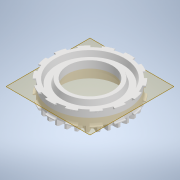
# Autodesk Inventor part: CAT_slave_wheel
Saved by Autodesk Inventor 2022 (Build 260153000, 153)
## iProperties
Created: 2024-07-28
Part Number: CAT_slave_wheel
Material: Типовые
Document SubType Name: Modeling
Designer: Капустяник Андрей
Density: 1 g/cm^3
Appearance: По умолчанию
Author: Капустяник Андрей
Autodesk Inventor part; units mm, degrees
ref_plane "YZ Plane" through (0, 0, 0) normal (1, 0, 0) x (0, 1, 0)
ref_plane "XZ Plane" through (0, 0, 0) normal (0, 1, 0) x (-1, 0, 0)
ref_plane "XY Plane" through (0, 0, 0) normal (0, 0, 1) x (1, 0, 0)
sketch "Эскиз1" plane through (0, 0, 0) normal (0, 1, 0) x (-1, 0, 0)
  circle A0 centre (0, 0) radius 35
  circle A1 centre (0, 0) radius 32
  circle A2 centre (0, 0) radius 18.5
  circle A3 centre (0, 0) radius 12.625
  circle A4 centre (0, 0) radius 18.6
  dimension "d0" = 70
  dimension "d1" = 3
  dimension "d2" = 37
  dimension "d3" = 25.25
  dimension "d4" = 37.2
  constraints: 5 centre point, 4 coincident
  measures "d0" diameter of A0
  measures "d1" radial gap between concentric circles of A0 A1
  measures "d2" diameter of A2
  measures "d3" diameter of A3
  measures "d4" diameter of A4
extrude "Выдавливание1" add sketch "Эскиз1" along normal blind 12 contours A1
sketch "Эскиз2" plane through (0, 0, 0) normal (0, -1, 0) x (1, 0, 0)
  circle A0 centre (0, 0) radius 32 projected
  circle A1 centre (0, 0) radius 18.6 projected
  circle A2 centre (-11.1467, 16) radius 3.5 projected
  circle A3 centre (-11.1467, 16) radius 6.5
  circle A4 centre (0, 0) radius 26
  dimension "d7" = 13
  constraints: 2 centre point, 2 coincident, 1 tangent
  measures "d7" diameter of A3
extrude "Выдавливание2" cut sketch "Эскиз2" against normal blind 5 contours A4 | A1 A2 A3 | A1 A2 picked at (-14.6701, 20.1761) picked at (-11.4582, 16.4471)
sketch "Эскиз3" plane through (0, 0, 0) normal (0, -1, 0) x (1, 0, 0)
  circle A0 centre (0, 0) radius 26
  circle A1 centre (0, 0) radius 32
  circle A2 centre (0, 0) radius 26
  circle A3 centre (0, 0) radius 18.6
  circle A4 centre (0, 0) radius 30
  spline S0 degree 3 poles (-0.9532, 24.4021) (-0.9433, 24.442) (-0.9236, 24.5218) (-0.8805, 24.6804) (-0.822, 24.8775) (-0.7447, 25.1117) (-0.661, 25.3437) (-0.5713, 25.5734) (-0.4759, 25.8008) (-0.3757, 26.0262) (-0.3047, 26.1745) (-0.2692, 26.2486) knots 0 0 0 0 0.062501 0.125002 0.25 0.374999 0.499998 0.624998 0.749999 0.875 1 1 1 1
  spline S1 degree 3 poles (0.9532, 24.4021) (0.9433, 24.442) (0.9236, 24.5218) (0.8805, 24.6804) (0.822, 24.8775) (0.7447, 25.1117) (0.661, 25.3437) (0.5713, 25.5734) (0.4759, 25.8008) (0.3757, 26.0262) (0.3047, 26.1745) (0.2692, 26.2486) knots 0 0 0 0 0.062501 0.125002 0.25 0.374999 0.499998 0.624998 0.749999 0.875 1 1 1 1
  circle A5 centre (0, 0) radius 26.25 construction
  circle A6 centre (0, 0) radius 23.4923 construction
  circle A7 centre (0, 0) radius 25 construction
  circle A8 centre (0, 0) radius 24.4207
  circle A9 centre (0, 0) radius 28.0793
  arc A10 (0.2692, 26.2486) -> (-0.2692, 26.2486) centre (0, 0) ccw
  point P0 (-0.9231, 24.5217)
  point P1 (-0.891, 24.6407)
  point P2 (-0.8208, 24.8771)
  point P3 (-0.7436, 25.1113)
  point P4 (-0.66, 25.3433)
  point P5 (-0.5703, 25.573)
  point P6 (-0.4751, 25.8005)
  point P7 (-0.3747, 26.0257)
  point P8 (0.9231, 24.5217)
  point P9 (0.891, 24.6407)
  point P10 (0.8208, 24.8771)
  point P11 (0.7436, 25.1113)
  point P12 (0.66, 25.3433)
  point P13 (0.5703, 25.573)
  point P14 (0.4751, 25.8005)
  point P15 (0.3747, 26.0257)
  dimension "d10" = 2
  constraints: 7 centre point, 6 point on circle, 47 other
  measures "d10" radial gap between concentric circles of A1 A4
extrude "Выдавливание3" add sketch "Эскиз3" along normal mid plane 10 contours A0 S0 A8 S1 | S1 A8 S0 A0 | A0 S0 A10 S1 | A4 | A9
sketch "Эскиз5" plane through (0, 0, 0) normal (1, 0, 0) x (0, 1, 0)
  line L0 (0, 32) -> (12, 32) projected
  line L1 (0, -32) -> (0, 32) projected
  line L2 (12, -32) -> (12, 32) projected
  line L3 (0, -32) -> (0, 32) projected
  line L4 (0, 32) -> (0, 34)
  line L5 (0, 34) -> (0.8, 34)
  spline S0 degree 4 poles (0.8, 34) (0.8, 33.0791) (1.2005, 31.7988) (2.191, 32) (3, 32) knots 0 0 0 0 0 1 1 1 1 1
  line L6 (0.8, 34) -> (0.8, 32)
  line L7 (0, 32) -> (3, 32)
  line L8 (12, -32) -> (12, 32) projected
  line L9 (12, 0) -> (0, 0)
  point P0 (1.5, 32.2689)
  point P1 (2.3311, 32)
  dimension "d18" = 2
  dimension "d19" = 0.8
  dimension "d20" = 3
  constraints: 10 end point, 3 perpendicular, 2 point on line, 2 vertical, 1 horizontal, 1 midpoint, 3 other
  measures "d18" distance of L3.end L4.end
  measures "d19" distance of L4.end L5.end
  measures "d20" distance of L3.end L7.end
revolve "Вращение1" add sketch "Эскиз5" angle 360 about axis through (0, 12, 0) along (0, -1, 0) contours L4 L5 L6 L0 | L6 S0 L0
fillet "Сопряжение1" radius 0.2 2 edges at (0, 0.8, -34) (0, 0, -34)
ref_plane "РабПлоскость1" through (0, 6, 0) normal (0, 1, 0) x (1, 0, 0)
mirror "Зеркальное отражение1" about plane through (0, 6, 0) normal (0, 1, 0) of "Вращение1", "Сопряжение1"
sketch "Эскиз6" plane through (0, 12, 0) normal (0, 1, 0) x (1, 0, 0)
  line L0 (0, 0) -> (-34, 0)
  circle A0 centre (0, 0) radius 34 projected
  line L1 (0, 0) -> (-33.8137, 3.554)
  circle A1 centre (0, 0) radius 32 projected
  circle A2 centre (0, 0) radius 32 projected
  line L2 (-33.8137, -3.554) -> (0, 0)
  point P0 (-25.0471, 7.8552)
  point P1 (0, -32)
  point P2 (0, -32)
  point P3 (-31.8247, -3.3449)
  point P4 (-31.8247, 3.3449)
  dimension "d24" = 12
  dimension "d25" = 6
  constraints: 6 end point, 3 point on circle, 1 horizontal, 1 vertical alignment, 1 other
  measures "d24" angle of L1 L2
  measures "d25" angle of L2 L0
extrude "Выдавливание5" cut sketch "Эскиз6" against normal blind 12 contours A1 L2 A0 L0 | L0 A0 L1 A1
pattern_circular "Круговой массив2" count 14 over 360 about axis through (0, 0, 0) along (0, 1, 0) of "Выдавливание5"
sketch "Эскиз7" plane through (0, 12, 0) normal (0, 1, 0) x (1, 0, 0)
  circle A0 centre (0, 0) radius 18.6 projected
  line L0 (-28.753, 17.7681) -> (-27.2218, 16.8219) projected
  arc A1 (-27.2218, 16.8219) -> (-30.1244, 10.7946) centre (0, 0) ccw projected
  line L1 (-30.1244, 10.7946) -> (-31.8189, 11.4018) projected
  arc A2 (-31.8189, 11.4018) -> (-33.6148, 3.5331) centre (0, 0) ccw projected
  line L2 (-33.6148, 3.5331) -> (-31.8247, 3.3449) projected
  arc A3 (-31.8247, 3.3449) -> (-31.8247, -3.3449) centre (0, 0) ccw projected
  line L3 (-31.8247, -3.3449) -> (-33.6148, -3.5331) projected
  arc A4 (-33.6148, -3.5331) -> (-31.8189, -11.4018) centre (0, 0) ccw projected
  line L4 (-31.8189, -11.4018) -> (-30.1244, -10.7946) projected
  arc A5 (-30.1244, -10.7946) -> (-27.2218, -16.8219) centre (0, 0) ccw projected
  line L5 (-27.2218, -16.8219) -> (-28.753, -17.7681) projected
  arc A6 (-28.753, -17.7681) -> (-23.7208, -24.0783) centre (0, 0) ccw projected
  line L6 (-23.7208, -24.0783) -> (-22.4575, -22.796) projected
  arc A7 (-22.4575, -22.796) -> (-17.2272, -26.9671) centre (0, 0) ccw projected
  line L7 (-17.2272, -26.9671) -> (-18.1963, -28.484) projected
  arc A8 (-18.1963, -28.484) -> (-10.9245, -31.9859) centre (0, 0) ccw projected
  line L8 (-10.9245, -31.9859) -> (-10.3427, -30.2825) projected
  arc A9 (-10.3427, -30.2825) -> (-3.8206, -31.7711) centre (0, 0) ccw projected
  line L9 (-3.8206, -31.7711) -> (-4.0355, -33.5582) projected
  arc A10 (-4.0355, -33.5582) -> (4.0355, -33.5582) centre (0, 0) ccw projected
  line L10 (4.0355, -33.5582) -> (3.8206, -31.7711) projected
  arc A11 (3.8206, -31.7711) -> (10.3427, -30.2825) centre (0, 0) ccw projected
  line L11 (10.3427, -30.2825) -> (10.9245, -31.9859) projected
  arc A12 (10.9245, -31.9859) -> (18.1963, -28.484) centre (0, 0) ccw projected
  line L12 (18.1963, -28.484) -> (17.2272, -26.9671) projected
  arc A13 (17.2272, -26.9671) -> (22.4575, -22.796) centre (0, 0) ccw projected
  line L13 (22.4575, -22.796) -> (23.7208, -24.0783) projected
  arc A14 (23.7208, -24.0783) -> (28.753, -17.7681) centre (0, 0) ccw projected
  line L14 (28.753, -17.7681) -> (27.2218, -16.8219) projected
  arc A15 (27.2218, -16.8219) -> (30.1244, -10.7946) centre (0, 0) ccw projected
  line L15 (30.1244, -10.7946) -> (31.8189, -11.4018) projected
  arc A16 (31.8189, -11.4018) -> (33.6148, -3.5331) centre (0, 0) ccw projected
  line L16 (33.6148, -3.5331) -> (31.8247, -3.3449) projected
  arc A17 (31.8247, -3.3449) -> (31.8247, 3.3449) centre (0, 0) ccw projected
  line L17 (31.8247, 3.3449) -> (33.6148, 3.5331) projected
  arc A18 (33.6148, 3.5331) -> (31.8189, 11.4018) centre (0, 0) ccw projected
  line L18 (31.8189, 11.4018) -> (30.1244, 10.7946) projected
  arc A19 (30.1244, 10.7946) -> (27.2218, 16.8219) centre (0, 0) ccw projected
  line L19 (27.2218, 16.8219) -> (28.753, 17.7681) projected
  arc A20 (28.753, 17.7681) -> (23.7208, 24.0783) centre (0, 0) ccw projected
  line L20 (23.7208, 24.0783) -> (22.4575, 22.796) projected
  arc A21 (22.4575, 22.796) -> (17.2272, 26.9671) centre (0, 0) ccw projected
  line L21 (17.2272, 26.9671) -> (18.1963, 28.484) projected
  arc A22 (18.1963, 28.484) -> (10.9245, 31.9859) centre (0, 0) ccw projected
  line L22 (10.9245, 31.9859) -> (10.3427, 30.2825) projected
  arc A23 (10.3427, 30.2825) -> (3.8206, 31.7711) centre (0, 0) ccw projected
  line L23 (3.8206, 31.7711) -> (4.0355, 33.5582) projected
  arc A24 (4.0355, 33.5582) -> (-4.0355, 33.5582) centre (0, 0) ccw projected
  line L24 (-4.0355, 33.5582) -> (-3.8206, 31.7711) projected
  arc A25 (-3.8206, 31.7711) -> (-10.3427, 30.2825) centre (0, 0) ccw projected
  line L25 (-10.3427, 30.2825) -> (-10.9245, 31.9859) projected
  arc A26 (-10.9245, 31.9859) -> (-18.1963, 28.484) centre (0, 0) ccw projected
  line L26 (-18.1963, 28.484) -> (-17.2272, 26.9671) projected
  arc A27 (-17.2272, 26.9671) -> (-22.4575, 22.796) centre (0, 0) ccw projected
  line L27 (-22.4575, 22.796) -> (-23.7208, 24.0783) projected
  arc A28 (-23.7208, 24.0783) -> (-28.753, 17.7681) centre (0, 0) ccw projected
  circle A29 centre (0, 0) radius 21.6
  circle A30 centre (0, 0) radius 32
  circle A31 centre (0, 0) radius 29
  dimension "d31" = 3
  dimension "d32" = 3
  constraints: 2 centre point, 1 coincident, 3 other
  measures "d31" radial gap between concentric circles of A0 A29
extrude "Выдавливание6" cut sketch "Эскиз7" against normal blind 4 contours A31
draft "НаклГрань1" angle 20 pull direction (0, 1, 0) faces at (21.53, 9.3333, 1.7381) fixed edges at (-21.6, 12, 0)
draft "НаклГрань2" angle 20 pull direction (0, 1, 0) faces at (28.906, 9.3333, 2.3335) fixed edges at (-29, 12, 0)
sketch "Эскиз8" plane through (0, -5, 0) normal (0, -1, 0) x (1, 0, 0)
  circle A0 centre (0, 0) radius 24.4207 projected
  circle A1 centre (0, 0) radius 30 projected
  spline S0 degree 3 poles (-2.6105, 31.8931) (-2.55, 31.7984) (-2.429, 31.6091) (-2.256, 31.3197) (-2.0897, 31.0266) (-1.931, 30.7291) (-1.7804, 30.4275) (-1.6387, 30.1217) (-1.5067, 29.8115) (-1.3853, 29.497) (-1.2943, 29.2312) (-1.2285, 29.0163) (-1.1831, 28.854) (-1.1418, 28.6906) (-1.1067, 28.5258) (-1.0789, 28.388) (-1.0493, 28.2796) (-1.0226, 28.1997) (-0.9926, 28.1209) (-0.9581, 28.044) (-0.9187, 27.9694) (-0.8741, 27.8979) (-0.8241, 27.8299) (-0.7687, 27.7663) (-0.7079, 27.7078) (-0.6415, 27.6557) (-0.5706, 27.6101) (-0.4961, 27.5705) (-0.4173, 27.5402) (-0.336, 27.5176) (-0.2528, 27.5029) (-0.1404, 27.4982) (0, 27.5012) (0.1404, 27.4982) (0.2528, 27.5029) (0.336, 27.5176) (0.4173, 27.5402) (0.4961, 27.5705) (0.5706, 27.6101) (0.6415, 27.6557) (0.7079, 27.7078) (0.7687, 27.7663) (0.8241, 27.8299) (0.8741, 27.8979) (0.9187, 27.9694) (0.9581, 28.044) (0.9926, 28.1209) (1.0226, 28.1997) (1.0493, 28.2796) (1.0789, 28.388) (1.1067, 28.5258) (1.1418, 28.6906) (1.1831, 28.854) (1.2285, 29.0163) (1.2943, 29.2312) (1.3853, 29.497) (1.5067, 29.8115) (1.6387, 30.1217) (1.7804, 30.4275) (1.931, 30.7291) (2.0897, 31.0266) (2.256, 31.3197) (2.429, 31.6091) (2.55, 31.7984) (2.6105, 31.8931) knots 0 0 0 0 0.033705 0.067411 0.101116 0.134821 0.168526 0.202231 0.235936 0.26964 0.303344 0.320197 0.33705 0.353902 0.370754 0.387605 0.396031 0.404457 0.412882 0.421308 0.429734 0.43816 0.446585 0.455011 0.463438 0.471862 0.480283 0.488707 0.497132 0.505555 0.51398 0.522403 0.539256 0.556109 0.564532 0.572957 0.58138 0.589805 0.598229 0.60665 0.615075 0.623501 0.631927 0.640352 0.648778 0.657205 0.66563 0.674055 0.682481 0.690907 0.707758 0.72461 0.741463 0.758315 0.775168 0.808872 0.842576 0.876281 0.909986 0.943691 0.977396 1.011101 1.044807 1.078512 1.078512 1.078512 1.078512
  circle A2 centre (0, 0) radius 27.5 construction
  circle A3 centre (0, 0) radius 28.1908 construction
  circle A4 centre (0, 0) radius 30 construction
  circle A5 centre (0, 0) radius 31.9997
  point P0 (-2.4304, 31.6082)
  point P1 (-2.2571, 31.3191)
  point P2 (-2.0909, 31.0258)
  point P3 (-1.9324, 30.7284)
  point P4 (-1.7819, 30.4268)
  point P5 (-1.6403, 30.1209)
  point P6 (-1.5084, 29.8108)
  point P7 (-1.3873, 29.4962)
  point P8 (-1.2784, 29.1773)
  point P9 (-1.2291, 29.0161)
  point P10 (-1.1838, 28.8538)
  point P11 (-1.1428, 28.6904)
  point P12 (-1.107, 28.5257)
  point P13 (-1.0709, 28.3611)
  point P14 (-1.0486, 28.2798)
  point P15 (-1.0221, 28.1999)
  point P16 (-0.9919, 28.1212)
  point P17 (-0.9573, 28.0444)
  point P18 (-0.9178, 27.9699)
  point P19 (-0.8732, 27.8985)
  point P20 (-0.8232, 27.8307)
  point P21 (-0.7678, 27.7672)
  point P22 (-0.7069, 27.7089)
  point P23 (-0.6407, 27.6567)
  point P24 (-0.57, 27.6111)
  point P25 (-0.4953, 27.572)
  point P26 (-0.4168, 27.5415)
  point P27 (-0.3357, 27.5189)
  point P28 (-0.2526, 27.5048)
  point P29 (-0.1685, 27.5)
  point P30 (0, 27.5)
  point P31 (0.1685, 27.5)
  point P32 (0.2526, 27.5048)
  point P33 (0.3357, 27.5189)
  point P34 (0.4168, 27.5415)
  point P35 (0.4953, 27.572)
  point P36 (0.57, 27.6111)
  point P37 (0.6407, 27.6567)
  point P38 (0.7069, 27.7089)
  point P39 (0.7678, 27.7672)
  point P40 (0.8232, 27.8307)
  point P41 (0.8732, 27.8985)
  point P42 (0.9178, 27.9699)
  point P43 (0.9573, 28.0444)
  point P44 (0.9919, 28.1212)
  point P45 (1.0221, 28.1999)
  point P46 (1.0486, 28.2798)
  point P47 (1.0709, 28.3611)
  point P48 (1.107, 28.5257)
  point P49 (1.1428, 28.6904)
  point P50 (1.1838, 28.8538)
  point P51 (1.2291, 29.0161)
  point P52 (1.2784, 29.1773)
  point P53 (1.3873, 29.4962)
  point P54 (1.5084, 29.8108)
  point P55 (1.6403, 30.1209)
  point P56 (1.7819, 30.4268)
  point P57 (1.9324, 30.7284)
  point P58 (2.0909, 31.0258)
  point P59 (2.2571, 31.3191)
  point P60 (2.4304, 31.6082)
  point P61 (-1.5699, 29.9589)
  point P62 (1.5699, 29.9589)
  constraints: 4 centre point, 2 point on circle, 131 other
extrude "Выдавливание7" add sketch "Эскиз8" against normal up to surface (5 mm away) contours A1 S0 A5 | S0 A1 | A1 S0 A5 picked at (0.1515, 28.9718)
sketch "Эскиз10" plane through (0, -5, 0) normal (0, -1, 0) x (1, 0, 0)
  spline S0 degree 3 poles (-2.6105, 31.8931) (-2.55, 31.7984) (-2.429, 31.6091) (-2.256, 31.3197) (-2.0897, 31.0266) (-1.931, 30.7291) (-1.7804, 30.4275) (-1.6387, 30.1217) (-1.5067, 29.8115) (-1.3853, 29.497) (-1.2943, 29.2312) (-1.2285, 29.0163) (-1.1831, 28.854) (-1.1418, 28.6906) (-1.1067, 28.5258) (-1.0789, 28.388) (-1.0493, 28.2796) (-1.0226, 28.1997) (-0.9926, 28.1209) (-0.9581, 28.044) (-0.9187, 27.9694) (-0.8741, 27.8979) (-0.8241, 27.8299) (-0.7687, 27.7663) (-0.7079, 27.7078) (-0.6415, 27.6557) (-0.5706, 27.6101) (-0.4961, 27.5705) (-0.4173, 27.5402) (-0.336, 27.5176) (-0.2528, 27.5029) (-0.1404, 27.4982) (0, 27.5012) (0.1404, 27.4982) (0.2528, 27.5029) (0.336, 27.5176) (0.4173, 27.5402) (0.4961, 27.5705) (0.5706, 27.6101) (0.6415, 27.6557) (0.7079, 27.7078) (0.7687, 27.7663) (0.8241, 27.8299) (0.8741, 27.8979) (0.9187, 27.9694) (0.9581, 28.044) (0.9926, 28.1209) (1.0226, 28.1997) (1.0493, 28.2796) (1.0789, 28.388) (1.1067, 28.5258) (1.1418, 28.6906) (1.1831, 28.854) (1.2285, 29.0163) (1.2943, 29.2312) (1.3853, 29.497) (1.5067, 29.8115) (1.6387, 30.1217) (1.7804, 30.4275) (1.931, 30.7291) (2.0897, 31.0266) (2.256, 31.3197) (2.429, 31.6091) (2.55, 31.7984) (2.6105, 31.8931) knots 0 0 0 0 0.033705 0.067411 0.101116 0.134821 0.168526 0.202231 0.235936 0.26964 0.303344 0.320197 0.33705 0.353902 0.370754 0.387605 0.396031 0.404457 0.412882 0.421308 0.429734 0.43816 0.446585 0.455011 0.463438 0.471862 0.480283 0.488707 0.497132 0.505555 0.51398 0.522403 0.539256 0.556109 0.564532 0.572957 0.58138 0.589805 0.598229 0.60665 0.615075 0.623501 0.631927 0.640352 0.648778 0.657205 0.66563 0.674055 0.682481 0.690907 0.707758 0.72461 0.741463 0.758315 0.775168 0.808872 0.842576 0.876281 0.909986 0.943691 0.977396 1.011101 1.044807 1.078512 1.078512 1.078512 1.078512
  circle A0 centre (0, 0) radius 27.5 construction
  circle A1 centre (0, 0) radius 28.1908 construction
  circle A2 centre (0, 0) radius 30 construction
  circle A3 centre (0, 0) radius 31.9997
  point P0 (-2.4304, 31.6082)
  point P1 (-2.2571, 31.3191)
  point P2 (-2.0909, 31.0258)
  point P3 (-1.9324, 30.7284)
  point P4 (-1.7819, 30.4268)
  point P5 (-1.6403, 30.1209)
  point P6 (-1.5084, 29.8108)
  point P7 (-1.3873, 29.4962)
  point P8 (-1.2784, 29.1773)
  point P9 (-1.2291, 29.0161)
  point P10 (-1.1838, 28.8538)
  point P11 (-1.1428, 28.6904)
  point P12 (-1.107, 28.5257)
  point P13 (-1.0709, 28.3611)
  point P14 (-1.0486, 28.2798)
  point P15 (-1.0221, 28.1999)
  point P16 (-0.9919, 28.1212)
  point P17 (-0.9573, 28.0444)
  point P18 (-0.9178, 27.9699)
  point P19 (-0.8732, 27.8985)
  point P20 (-0.8232, 27.8307)
  point P21 (-0.7678, 27.7672)
  point P22 (-0.7069, 27.7089)
  point P23 (-0.6407, 27.6567)
  point P24 (-0.57, 27.6111)
  point P25 (-0.4953, 27.572)
  point P26 (-0.4168, 27.5415)
  point P27 (-0.3357, 27.5189)
  point P28 (-0.2526, 27.5048)
  point P29 (-0.1685, 27.5)
  point P30 (0, 27.5)
  point P31 (0.1685, 27.5)
  point P32 (0.2526, 27.5048)
  point P33 (0.3357, 27.5189)
  point P34 (0.4168, 27.5415)
  point P35 (0.4953, 27.572)
  point P36 (0.57, 27.6111)
  point P37 (0.6407, 27.6567)
  point P38 (0.7069, 27.7089)
  point P39 (0.7678, 27.7672)
  point P40 (0.8232, 27.8307)
  point P41 (0.8732, 27.8985)
  point P42 (0.9178, 27.9699)
  point P43 (0.9573, 28.0444)
  point P44 (0.9919, 28.1212)
  point P45 (1.0221, 28.1999)
  point P46 (1.0486, 28.2798)
  point P47 (1.0709, 28.3611)
  point P48 (1.107, 28.5257)
  point P49 (1.1428, 28.6904)
  point P50 (1.1838, 28.8538)
  point P51 (1.2291, 29.0161)
  point P52 (1.2784, 29.1773)
  point P53 (1.3873, 29.4962)
  point P54 (1.5084, 29.8108)
  point P55 (1.6403, 30.1209)
  point P56 (1.7819, 30.4268)
  point P57 (1.9324, 30.7284)
  point P58 (2.0909, 31.0258)
  point P59 (2.2571, 31.3191)
  point P60 (2.4304, 31.6082)
  constraints: 4 centre point, 2 point on circle, 131 other
extrude "Выдавливание8" cut sketch "Эскиз10" against normal up to surface (5 mm away) contours A3 S0 picked at (-0.1928, 30.4433)
chamfer "Фаска1" distance 0.5 angle 45 2 edges at (23.5321, -5, 21.6846) (-21.6846, -5, -23.5321)
pattern_circular "Круговой массив3" count 30 over 360 about axis through (0, 0, 0) along (0, 1, 0) of "Выдавливание8"
sketch "Эскиз11" plane through (0, -5, 0) normal (0, -1, 0) x (1, 0, 0)
  circle A0 centre (0, 0) radius 24.4207 projected
  circle A1 centre (0, 0) radius 18.6 projected
  circle A2 centre (0, 0) radius 24
  dimension "d47" = 48
  constraints: 1 centre point, 1 coincident
  measures "d47" diameter of A2
extrude "Выдавливание9" add sketch "Эскиз11" against normal up to surface (10 mm away) contours A0
chamfer "Фаска2" distance 4 angle 45 1 edges at (-24, 5, 0)
sketch "Эскиз12" plane through (0, 5, 0) normal (0, -1, 0) x (1, 0, 0)
  spline S0 degree 3 poles (-3.0227, 26.0754) (-2.9839, 26.0151) (-2.9328, 25.9363) (-2.8735, 25.8407) knots 0 0 0 0 1 1 1 1
  arc A0 (-3.0227, 26.0754) -> (-3.5569, 26.0079) centre (0, 0) ccw
  spline S1 degree 3 poles (-3.6431, 25.7435) (-3.6095, 25.8508) (-3.5795, 25.9399) (-3.5569, 26.0079) knots 0 0 0 0 1 1 1 1
  spline S2 degree 3 poles (-6.267, 25.4909) (-6.2209, 25.436) (-6.1603, 25.3642) (-6.0896, 25.2768) knots 0 0 0 0 1 1 1 1
  arc A1 (-6.267, 25.4909) -> (-6.7885, 25.357) centre (0, 0) ccw
  spline S3 degree 3 poles (-6.8409, 25.0839) (-6.821, 25.1946) (-6.8024, 25.2867) (-6.7885, 25.357) knots 0 0 0 0 1 1 1 1
  spline S4 degree 3 poles (-9.4125, 24.5045) (-9.3599, 24.4557) (-9.2907, 24.3921) (-9.2096, 24.3143) knots 0 0 0 0 1 1 1 1
  arc A2 (-9.4125, 24.5045) -> (-9.9131, 24.3062) centre (0, 0) ccw
  spline S5 degree 3 poles (-9.9308, 24.0287) (-9.9249, 24.1411) (-9.9181, 24.2347) (-9.9131, 24.3062) knots 0 0 0 0 1 1 1 1
  spline S6 degree 3 poles (-12.4095, 23.1315) (-12.3512, 23.0898) (-12.2746, 23.0354) (-12.1843, 22.9683) knots 0 0 0 0 1 1 1 1
  arc A3 (-12.4095, 23.1315) -> (-12.8813, 22.8721) centre (0, 0) ccw
  spline S7 degree 3 poles (-12.8641, 22.5946) (-12.8723, 22.7068) (-12.8773, 22.8006) (-12.8813, 22.8721) knots 0 0 0 0 1 1 1 1
  spline S8 degree 3 poles (-15.2108, 21.3938) (-15.1477, 21.3597) (-15.0649, 21.3153) (-14.967, 21.2601) knots 0 0 0 0 1 1 1 1
  arc A4 (-15.2108, 21.3938) -> (-15.6464, 21.0773) centre (0, 0) ccw
  spline S9 degree 3 poles (-15.5945, 20.8041) (-15.6167, 20.9144) (-15.6334, 21.0068) (-15.6464, 21.0773) knots 0 0 0 0 1 1 1 1
  spline S10 degree 3 poles (-17.7722, 19.3187) (-17.7053, 19.2928) (-17.6177, 19.2591) (-17.5135, 19.2166) knots 0 0 0 0 1 1 1 1
  arc A5 (-17.7722, 19.3187) -> (-18.1647, 18.9501) centre (0, 0) ccw
  spline S11 degree 3 poles (-18.079, 18.6856) (-18.1149, 18.7922) (-18.143, 18.8818) (-18.1647, 18.9501) knots 0 0 0 0 1 1 1 1
  spline S12 degree 3 poles (-20.0533, 16.9389) (-19.9837, 16.9216) (-19.8925, 16.8992) (-19.7839, 16.87) knots 0 0 0 0 1 1 1 1
  arc A6 (-20.0533, 16.9389) -> (-20.3965, 16.5241) centre (0, 0) ccw
  spline S13 degree 3 poles (-20.2783, 16.2724) (-20.3273, 16.3736) (-20.3664, 16.459) (-20.3965, 16.5241) knots 0 0 0 0 1 1 1 1
  spline S14 degree 3 poles (-22.0182, 14.292) (-21.947, 14.2835) (-21.8537, 14.2727) (-21.7423, 14.2574) knots 0 0 0 0 1 1 1 1
  arc A7 (-22.0182, 14.292) -> (-22.3067, 13.8374) centre (0, 0) ccw
  spline S15 degree 3 poles (-22.1579, 13.6025) (-22.2192, 13.6968) (-22.2687, 13.7766) (-22.3067, 13.8374) knots 0 0 0 0 1 1 1 1
  spline S16 degree 3 poles (-23.6358, 11.4197) (-23.5641, 11.4202) (-23.4702, 11.4212) (-23.3578, 11.4199) knots 0 0 0 0 1 1 1 1
  arc A8 (-23.6358, 11.4197) -> (-23.8651, 10.9325) centre (0, 0) ccw
  spline S17 degree 3 poles (-23.688, 10.7181) (-23.7606, 10.804) (-23.8198, 10.877) (-23.8651, 10.9325) knots 0 0 0 0 1 1 1 1
  spline S18 degree 3 poles (-24.8807, 8.3673) (-24.8097, 8.3768) (-24.7166, 8.3895) (-24.6049, 8.4024) knots 0 0 0 0 1 1 1 1
  arc A9 (-24.8807, 8.3673) -> (-25.0471, 7.8552) centre (0, 0) ccw
  spline S19 degree 3 poles (-24.8446, 7.6647) (-24.9274, 7.7408) (-24.9952, 7.8058) (-25.0471, 7.8552) knots 0 0 0 0 1 1 1 1
  spline S20 degree 3 poles (-25.7332, 5.1829) (-25.6639, 5.2012) (-25.5732, 5.2255) (-25.464, 5.2523) knots 0 0 0 0 1 1 1 1
  arc A10 (-25.7332, 5.1829) -> (-25.8341, 4.6541) centre (0, 0) ccw
  spline S21 degree 3 poles (-25.6093, 4.4904) (-25.701, 4.5555) (-25.7764, 4.6115) (-25.8341, 4.6541) knots 0 0 0 0 1 1 1 1
  spline S22 degree 3 poles (-26.1799, 1.9168) (-26.1134, 1.9437) (-26.0265, 1.9792) (-25.9215, 2.0194) knots 0 0 0 0 1 1 1 1
  arc A11 (-26.1799, 1.9168) -> (-26.2137, 1.3795) centre (0, 0) ccw
  spline S23 degree 3 poles (-25.9702, 1.2453) (-26.0693, 1.2984) (-26.1511, 1.3445) (-26.2137, 1.3795) knots 0 0 0 0 1 1 1 1
  spline S24 degree 3 poles (-26.2137, -1.3795) (-26.1511, -1.3445) (-26.0693, -1.2984) (-25.9702, -1.2453) knots 0 0 0 0 1 1 1 1
  arc A12 (-26.2137, -1.3795) -> (-26.1799, -1.9168) centre (0, 0) ccw
  spline S25 degree 3 poles (-25.9215, -2.0194) (-26.0265, -1.9792) (-26.1134, -1.9437) (-26.1799, -1.9168) knots 0 0 0 0 1 1 1 1
  spline S26 degree 3 poles (-25.8341, -4.6541) (-25.7764, -4.6115) (-25.701, -4.5555) (-25.6093, -4.4904) knots 0 0 0 0 1 1 1 1
  arc A13 (-25.8341, -4.6541) -> (-25.7332, -5.1829) centre (0, 0) ccw
  spline S27 degree 3 poles (-25.464, -5.2523) (-25.5732, -5.2255) (-25.6639, -5.2012) (-25.7332, -5.1829) knots 0 0 0 0 1 1 1 1
  spline S28 degree 3 poles (-25.0471, -7.8552) (-24.9952, -7.8058) (-24.9274, -7.7408) (-24.8446, -7.6647) knots 0 0 0 0 1 1 1 1
  arc A14 (-25.0471, -7.8552) -> (-24.8807, -8.3673) centre (0, 0) ccw
  spline S29 degree 3 poles (-24.6049, -8.4024) (-24.7166, -8.3895) (-24.8097, -8.3768) (-24.8807, -8.3673) knots 0 0 0 0 1 1 1 1
  spline S30 degree 3 poles (-23.8651, -10.9325) (-23.8198, -10.877) (-23.7606, -10.804) (-23.688, -10.7181) knots 0 0 0 0 1 1 1 1
  arc A15 (-23.8651, -10.9325) -> (-23.6358, -11.4197) centre (0, 0) ccw
  spline S31 degree 3 poles (-23.3578, -11.4199) (-23.4702, -11.4212) (-23.5641, -11.4202) (-23.6358, -11.4197) knots 0 0 0 0 1 1 1 1
  spline S32 degree 3 poles (-22.3067, -13.8374) (-22.2687, -13.7766) (-22.2192, -13.6968) (-22.1579, -13.6025) knots 0 0 0 0 1 1 1 1
  arc A16 (-22.3067, -13.8374) -> (-22.0182, -14.292) centre (0, 0) ccw
  spline S33 degree 3 poles (-21.7423, -14.2574) (-21.8537, -14.2727) (-21.947, -14.2835) (-22.0182, -14.292) knots 0 0 0 0 1 1 1 1
  spline S34 degree 3 poles (-20.3965, -16.5241) (-20.3664, -16.459) (-20.3273, -16.3736) (-20.2783, -16.2724) knots 0 0 0 0 1 1 1 1
  arc A17 (-20.3965, -16.5241) -> (-20.0533, -16.9389) centre (0, 0) ccw
  spline S35 degree 3 poles (-19.7839, -16.87) (-19.8925, -16.8992) (-19.9837, -16.9216) (-20.0533, -16.9389) knots 0 0 0 0 1 1 1 1
  spline S36 degree 3 poles (-18.1647, -18.9501) (-18.143, -18.8818) (-18.1149, -18.7922) (-18.079, -18.6856) knots 0 0 0 0 1 1 1 1
  arc A18 (-18.1647, -18.9501) -> (-17.7722, -19.3187) centre (0, 0) ccw
  spline S37 degree 3 poles (-17.5135, -19.2166) (-17.6177, -19.2591) (-17.7053, -19.2928) (-17.7722, -19.3187) knots 0 0 0 0 1 1 1 1
  spline S38 degree 3 poles (-15.6464, -21.0773) (-15.6334, -21.0068) (-15.6167, -20.9144) (-15.5945, -20.8041) knots 0 0 0 0 1 1 1 1
  arc A19 (-15.6464, -21.0773) -> (-15.2108, -21.3938) centre (0, 0) ccw
  spline S39 degree 3 poles (-14.967, -21.2601) (-15.0649, -21.3153) (-15.1477, -21.3597) (-15.2108, -21.3938) knots 0 0 0 0 1 1 1 1
  spline S40 degree 3 poles (-12.8813, -22.8721) (-12.8773, -22.8006) (-12.8723, -22.7068) (-12.8641, -22.5946) knots 0 0 0 0 1 1 1 1
  arc A20 (-12.8813, -22.8721) -> (-12.4095, -23.1315) centre (0, 0) ccw
  spline S41 degree 3 poles (-12.1843, -22.9683) (-12.2746, -23.0354) (-12.3512, -23.0898) (-12.4095, -23.1315) knots 0 0 0 0 1 1 1 1
  spline S42 degree 3 poles (-9.9131, -24.3062) (-9.9181, -24.2347) (-9.9249, -24.1411) (-9.9308, -24.0287) knots 0 0 0 0 1 1 1 1
  arc A21 (-9.9131, -24.3062) -> (-9.4125, -24.5045) centre (0, 0) ccw
  spline S43 degree 3 poles (-9.2096, -24.3143) (-9.2907, -24.3921) (-9.3599, -24.4557) (-9.4125, -24.5045) knots 0 0 0 0 1 1 1 1
  spline S44 degree 3 poles (-6.7885, -25.357) (-6.8024, -25.2867) (-6.821, -25.1946) (-6.8409, -25.0839) knots 0 0 0 0 1 1 1 1
  arc A22 (-6.7885, -25.357) -> (-6.267, -25.4909) centre (0, 0) ccw
  spline S45 degree 3 poles (-6.0896, -25.2768) (-6.1603, -25.3642) (-6.2209, -25.436) (-6.267, -25.4909) knots 0 0 0 0 1 1 1 1
  spline S46 degree 3 poles (-3.5569, -26.0079) (-3.5795, -25.9399) (-3.6095, -25.8508) (-3.6431, -25.7435) knots 0 0 0 0 1 1 1 1
  arc A23 (-3.5569, -26.0079) -> (-3.0227, -26.0754) centre (0, 0) ccw
  spline S47 degree 3 poles (-2.8735, -25.8407) (-2.9328, -25.9363) (-2.9839, -26.0151) (-3.0227, -26.0754) knots 0 0 0 0 1 1 1 1
  spline S48 degree 3 poles (-0.2692, -26.2486) (-0.3002, -26.184) (-0.341, -26.0994) (-0.3878, -25.9971) knots 0 0 0 0 1 1 1 1
  arc A24 (-0.2692, -26.2486) -> (0.2692, -26.2486) centre (0, 0) ccw
  spline S49 degree 3 poles (0.3878, -25.9971) (0.341, -26.0994) (0.3002, -26.184) (0.2692, -26.2486) knots 0 0 0 0 1 1 1 1
  spline S50 degree 3 poles (3.0227, -26.0754) (2.9839, -26.0151) (2.9328, -25.9363) (2.8735, -25.8407) knots 0 0 0 0 1 1 1 1
  arc A25 (3.0227, -26.0754) -> (3.5569, -26.0079) centre (0, 0) ccw
  spline S51 degree 3 poles (3.6431, -25.7435) (3.6095, -25.8508) (3.5795, -25.9399) (3.5569, -26.0079) knots 0 0 0 0 1 1 1 1
  spline S52 degree 3 poles (6.267, -25.4909) (6.2209, -25.436) (6.1603, -25.3642) (6.0896, -25.2768) knots 0 0 0 0 1 1 1 1
  arc A26 (6.267, -25.4909) -> (6.7885, -25.357) centre (0, 0) ccw
  spline S53 degree 3 poles (6.8409, -25.0839) (6.821, -25.1946) (6.8024, -25.2867) (6.7885, -25.357) knots 0 0 0 0 1 1 1 1
  spline S54 degree 3 poles (9.4125, -24.5045) (9.3599, -24.4557) (9.2907, -24.3921) (9.2096, -24.3143) knots 0 0 0 0 1 1 1 1
  arc A27 (9.4125, -24.5045) -> (9.9131, -24.3062) centre (0, 0) ccw
  spline S55 degree 3 poles (9.9308, -24.0287) (9.9249, -24.1411) (9.9181, -24.2347) (9.9131, -24.3062) knots 0 0 0 0 1 1 1 1
  spline S56 degree 3 poles (12.4095, -23.1315) (12.3512, -23.0898) (12.2746, -23.0354) (12.1843, -22.9683) knots 0 0 0 0 1 1 1 1
  arc A28 (12.4095, -23.1315) -> (12.8813, -22.8721) centre (0, 0) ccw
  spline S57 degree 3 poles (12.8641, -22.5946) (12.8723, -22.7068) (12.8773, -22.8006) (12.8813, -22.8721) knots 0 0 0 0 1 1 1 1
  spline S58 degree 3 poles (15.2108, -21.3938) (15.1477, -21.3597) (15.0649, -21.3153) (14.967, -21.2601) knots 0 0 0 0 1 1 1 1
  arc A29 (15.2108, -21.3938) -> (15.6464, -21.0773) centre (0, 0) ccw
  spline S59 degree 3 poles (15.5945, -20.8041) (15.6167, -20.9144) (15.6334, -21.0068) (15.6464, -21.0773) knots 0 0 0 0 1 1 1 1
  spline S60 degree 3 poles (17.7722, -19.3187) (17.7053, -19.2928) (17.6177, -19.2591) (17.5135, -19.2166) knots 0 0 0 0 1 1 1 1
  arc A30 (17.7722, -19.3187) -> (18.1647, -18.9501) centre (0, 0) ccw
  spline S61 degree 3 poles (18.079, -18.6856) (18.1149, -18.7922) (18.143, -18.8818) (18.1647, -18.9501) knots 0 0 0 0 1 1 1 1
  spline S62 degree 3 poles (20.0533, -16.9389) (19.9837, -16.9216) (19.8925, -16.8992) (19.7839, -16.87) knots 0 0 0 0 1 1 1 1
  arc A31 (20.0533, -16.9389) -> (20.3965, -16.5241) centre (0, 0) ccw
  spline S63 degree 3 poles (20.2783, -16.2724) (20.3273, -16.3736) (20.3664, -16.459) (20.3965, -16.5241) knots 0 0 0 0 1 1 1 1
  spline S64 degree 3 poles (22.0182, -14.292) (21.947, -14.2835) (21.8537, -14.2727) (21.7423, -14.2574) knots 0 0 0 0 1 1 1 1
  arc A32 (22.0182, -14.292) -> (22.3067, -13.8374) centre (0, 0) ccw
  spline S65 degree 3 poles (22.1579, -13.6025) (22.2192, -13.6968) (22.2687, -13.7766) (22.3067, -13.8374) knots 0 0 0 0 1 1 1 1
  spline S66 degree 3 poles (23.6358, -11.4197) (23.5641, -11.4202) (23.4702, -11.4212) (23.3578, -11.4199) knots 0 0 0 0 1 1 1 1
  arc A33 (23.6358, -11.4197) -> (23.8651, -10.9325) centre (0, 0) ccw
  spline S67 degree 3 poles (23.688, -10.7181) (23.7606, -10.804) (23.8198, -10.877) (23.8651, -10.9325) knots 0 0 0 0 1 1 1 1
  spline S68 degree 3 poles (24.8807, -8.3673) (24.8097, -8.3768) (24.7166, -8.3895) (24.6049, -8.4024) knots 0 0 0 0 1 1 1 1
  arc A34 (24.8807, -8.3673) -> (25.0471, -7.8552) centre (0, 0) ccw
  spline S69 degree 3 poles (24.8446, -7.6647) (24.9274, -7.7408) (24.9952, -7.8058) (25.0471, -7.8552) knots 0 0 0 0 1 1 1 1
  spline S70 degree 3 poles (25.7332, -5.1829) (25.6639, -5.2012) (25.5732, -5.2255) (25.464, -5.2523) knots 0 0 0 0 1 1 1 1
  arc A35 (25.7332, -5.1829) -> (25.8341, -4.6541) centre (0, 0) ccw
  spline S71 degree 3 poles (25.6093, -4.4904) (25.701, -4.5555) (25.7764, -4.6115) (25.8341, -4.6541) knots 0 0 0 0 1 1 1 1
  spline S72 degree 3 poles (26.1799, -1.9168) (26.1134, -1.9437) (26.0265, -1.9792) (25.9215, -2.0194) knots 0 0 0 0 1 1 1 1
  arc A36 (26.1799, -1.9168) -> (26.2137, -1.3795) centre (0, 0) ccw
  spline S73 degree 3 poles (25.9702, -1.2453) (26.0693, -1.2984) (26.1511, -1.3445) (26.2137, -1.3795) knots 0 0 0 0 1 1 1 1
  spline S74 degree 3 poles (26.2137, 1.3795) (26.1511, 1.3445) (26.0693, 1.2984) (25.9702, 1.2453) knots 0 0 0 0 1 1 1 1
  arc A37 (26.2137, 1.3795) -> (26.1799, 1.9168) centre (0, 0) ccw
  spline S75 degree 3 poles (25.9215, 2.0194) (26.0265, 1.9792) (26.1134, 1.9437) (26.1799, 1.9168) knots 0 0 0 0 1 1 1 1
  spline S76 degree 3 poles (25.8341, 4.6541) (25.7764, 4.6115) (25.701, 4.5555) (25.6093, 4.4904) knots 0 0 0 0 1 1 1 1
  arc A38 (25.8341, 4.6541) -> (25.7332, 5.1829) centre (0, 0) ccw
  spline S77 degree 3 poles (25.464, 5.2523) (25.5732, 5.2255) (25.6639, 5.2012) (25.7332, 5.1829) knots 0 0 0 0 1 1 1 1
  spline S78 degree 3 poles (25.0471, 7.8552) (24.9952, 7.8058) (24.9274, 7.7408) (24.8446, 7.6647) knots 0 0 0 0 1 1 1 1
  arc A39 (25.0471, 7.8552) -> (24.8807, 8.3673) centre (0, 0) ccw
  spline S79 degree 3 poles (24.6049, 8.4024) (24.7166, 8.3895) (24.8097, 8.3768) (24.8807, 8.3673) knots 0 0 0 0 1 1 1 1
  spline S80 degree 3 poles (23.8651, 10.9325) (23.8198, 10.877) (23.7606, 10.804) (23.688, 10.7181) knots 0 0 0 0 1 1 1 1
  arc A40 (23.8651, 10.9325) -> (23.6358, 11.4197) centre (0, 0) ccw
  spline S81 degree 3 poles (23.3578, 11.4199) (23.4702, 11.4212) (23.5641, 11.4202) (23.6358, 11.4197) knots 0 0 0 0 1 1 1 1
  spline S82 degree 3 poles (22.3067, 13.8374) (22.2687, 13.7766) (22.2192, 13.6968) (22.1579, 13.6025) knots 0 0 0 0 1 1 1 1
  arc A41 (22.3067, 13.8374) -> (22.0182, 14.292) centre (0, 0) ccw
  spline S83 degree 3 poles (21.7423, 14.2574) (21.8537, 14.2727) (21.947, 14.2835) (22.0182, 14.292) knots 0 0 0 0 1 1 1 1
  spline S84 degree 3 poles (20.3965, 16.5241) (20.3664, 16.459) (20.3273, 16.3736) (20.2783, 16.2724) knots 0 0 0 0 1 1 1 1
  arc A42 (20.3965, 16.5241) -> (20.0533, 16.9389) centre (0, 0) ccw
  spline S85 degree 3 poles (19.7839, 16.87) (19.8925, 16.8992) (19.9837, 16.9216) (20.0533, 16.9389) knots 0 0 0 0 1 1 1 1
  spline S86 degree 3 poles (18.1647, 18.9501) (18.143, 18.8818) (18.1149, 18.7922) (18.079, 18.6856) knots 0 0 0 0 1 1 1 1
  arc A43 (18.1647, 18.9501) -> (17.7722, 19.3187) centre (0, 0) ccw
  spline S87 degree 3 poles (17.5135, 19.2166) (17.6177, 19.2591) (17.7053, 19.2928) (17.7722, 19.3187) knots 0 0 0 0 1 1 1 1
  spline S88 degree 3 poles (15.6464, 21.0773) (15.6334, 21.0068) (15.6167, 20.9144) (15.5945, 20.8041) knots 0 0 0 0 1 1 1 1
  arc A44 (15.6464, 21.0773) -> (15.2108, 21.3938) centre (0, 0) ccw
  spline S89 degree 3 poles (14.967, 21.2601) (15.0649, 21.3153) (15.1477, 21.3597) (15.2108, 21.3938) knots 0 0 0 0 1 1 1 1
  spline S90 degree 3 poles (12.8813, 22.8721) (12.8773, 22.8006) (12.8723, 22.7068) (12.8641, 22.5946) knots 0 0 0 0 1 1 1 1
  arc A45 (12.8813, 22.8721) -> (12.4095, 23.1315) centre (0, 0) ccw
  spline S91 degree 3 poles (12.1843, 22.9683) (12.2746, 23.0354) (12.3512, 23.0898) (12.4095, 23.1315) knots 0 0 0 0 1 1 1 1
  spline S92 degree 3 poles (9.9131, 24.3062) (9.9181, 24.2347) (9.9249, 24.1411) (9.9308, 24.0287) knots 0 0 0 0 1 1 1 1
  arc A46 (9.9131, 24.3062) -> (9.4125, 24.5045) centre (0, 0) ccw
  spline S93 degree 3 poles (9.2096, 24.3143) (9.2907, 24.3921) (9.3599, 24.4557) (9.4125, 24.5045) knots 0 0 0 0 1 1 1 1
  spline S94 degree 3 poles (6.7885, 25.357) (6.8024, 25.2867) (6.821, 25.1946) (6.8409, 25.0839) knots 0 0 0 0 1 1 1 1
  arc A47 (6.7885, 25.357) -> (6.267, 25.4909) centre (0, 0) ccw
  spline S95 degree 3 poles (6.0896, 25.2768) (6.1603, 25.3642) (6.2209, 25.436) (6.267, 25.4909) knots 0 0 0 0 1 1 1 1
  spline S96 degree 3 poles (3.5569, 26.0079) (3.5795, 25.9399) (3.6095, 25.8508) (3.6431, 25.7435) knots 0 0 0 0 1 1 1 1
  arc A48 (3.5569, 26.0079) -> (3.0227, 26.0754) centre (0, 0) ccw
  spline S97 degree 3 poles (2.8735, 25.8407) (2.9328, 25.9363) (2.9839, 26.0151) (3.0227, 26.0754) knots 0 0 0 0 1 1 1 1
  spline S98 degree 3 poles (0.2692, 26.2486) (0.3002, 26.184) (0.341, 26.0994) (0.3878, 25.9971) knots 0 0 0 0 1 1 1 1
  arc A49 (0.2692, 26.2486) -> (-0.2692, 26.2486) centre (0, 0) ccw
  spline S99 degree 3 poles (-0.3878, 25.9971) (-0.341, 26.0994) (-0.3002, 26.184) (-0.2692, 26.2486) knots 0 0 0 0 1 1 1 1
  circle A50 centre (0, 0) radius 18.6
  circle A51 centre (0, 0) radius 19.6
  arc A52 (2.8735, 25.8407) -> (0.3878, 25.9971) centre (0, 0) ccw
  arc A53 (-0.3878, 25.9971) -> (-2.8735, 25.8407) centre (0, 0) ccw
  arc A54 (-3.6431, 25.7435) -> (-6.0896, 25.2768) centre (0, 0) ccw
  arc A55 (-6.8409, 25.0839) -> (-9.2096, 24.3143) centre (0, 0) ccw
  arc A56 (-9.9308, 24.0287) -> (-12.1843, 22.9683) centre (0, 0) ccw
  arc A57 (-12.8641, 22.5946) -> (-14.967, 21.2601) centre (0, 0) ccw
  arc A58 (-15.5945, 20.8041) -> (-17.5135, 19.2166) centre (0, 0) ccw
  arc A59 (-18.079, 18.6856) -> (-19.7839, 16.87) centre (0, 0) ccw
  arc A60 (-20.2783, 16.2724) -> (-21.7423, 14.2574) centre (0, 0) ccw
  arc A61 (-22.1579, 13.6025) -> (-23.3578, 11.4199) centre (0, 0) ccw
  arc A62 (-23.688, 10.7181) -> (-24.6049, 8.4024) centre (0, 0) ccw
  arc A63 (-24.8446, 7.6647) -> (-25.464, 5.2523) centre (0, 0) ccw
  arc A64 (-25.6093, 4.4904) -> (-25.9215, 2.0194) centre (0, 0) ccw
  arc A65 (-25.9702, 1.2453) -> (-25.9702, -1.2453) centre (0, 0) ccw
  arc A66 (-25.9215, -2.0194) -> (-25.6093, -4.4904) centre (0, 0) ccw
  arc A67 (-25.464, -5.2523) -> (-24.8446, -7.6647) centre (0, 0) ccw
  arc A68 (-24.6049, -8.4024) -> (-23.688, -10.7181) centre (0, 0) ccw
  arc A69 (-23.3578, -11.4199) -> (-22.1579, -13.6025) centre (0, 0) ccw
  arc A70 (-21.7423, -14.2574) -> (-20.2783, -16.2724) centre (0, 0) ccw
  arc A71 (-19.7839, -16.87) -> (-18.079, -18.6856) centre (0, 0) ccw
  arc A72 (-17.5135, -19.2166) -> (-15.5945, -20.8041) centre (0, 0) ccw
  arc A73 (-14.967, -21.2601) -> (-12.8641, -22.5946) centre (0, 0) ccw
  arc A74 (-12.1843, -22.9683) -> (-9.9308, -24.0287) centre (0, 0) ccw
  arc A75 (-9.2096, -24.3143) -> (-6.8409, -25.0839) centre (0, 0) ccw
  arc A76 (-6.0896, -25.2768) -> (-3.6431, -25.7435) centre (0, 0) ccw
  arc A77 (-2.8735, -25.8407) -> (-0.3878, -25.9971) centre (0, 0) ccw
  arc A78 (0.3878, -25.9971) -> (2.8735, -25.8407) centre (0, 0) ccw
  arc A79 (3.6431, -25.7435) -> (6.0896, -25.2768) centre (0, 0) ccw
  arc A80 (6.8409, -25.0839) -> (9.2096, -24.3143) centre (0, 0) ccw
  arc A81 (9.9308, -24.0287) -> (12.1843, -22.9683) centre (0, 0) ccw
  arc A82 (12.8641, -22.5946) -> (14.967, -21.2601) centre (0, 0) ccw
  arc A83 (15.5945, -20.8041) -> (17.5135, -19.2166) centre (0, 0) ccw
  arc A84 (18.079, -18.6856) -> (19.7839, -16.87) centre (0, 0) ccw
  arc A85 (20.2783, -16.2724) -> (21.7423, -14.2574) centre (0, 0) ccw
  arc A86 (22.1579, -13.6025) -> (23.3578, -11.4199) centre (0, 0) ccw
  arc A87 (23.688, -10.7181) -> (24.6049, -8.4024) centre (0, 0) ccw
  arc A88 (24.8446, -7.6647) -> (25.464, -5.2523) centre (0, 0) ccw
  arc A89 (25.6093, -4.4904) -> (25.9215, -2.0194) centre (0, 0) ccw
  arc A90 (25.9702, -1.2453) -> (25.9702, 1.2453) centre (0, 0) ccw
  arc A91 (25.9215, 2.0194) -> (25.6093, 4.4904) centre (0, 0) ccw
  arc A92 (25.464, 5.2523) -> (24.8446, 7.6647) centre (0, 0) ccw
  arc A93 (24.6049, 8.4024) -> (23.688, 10.7181) centre (0, 0) ccw
  arc A94 (23.3578, 11.4199) -> (22.1579, 13.6025) centre (0, 0) ccw
  arc A95 (21.7423, 14.2574) -> (20.2783, 16.2724) centre (0, 0) ccw
  arc A96 (19.7839, 16.87) -> (18.079, 18.6856) centre (0, 0) ccw
  arc A97 (17.5135, 19.2166) -> (15.5945, 20.8041) centre (0, 0) ccw
  arc A98 (14.967, 21.2601) -> (12.8641, 22.5946) centre (0, 0) ccw
  arc A99 (12.1843, 22.9683) -> (9.9308, 24.0287) centre (0, 0) ccw
  arc A100 (9.2096, 24.3143) -> (6.8409, 25.0839) centre (0, 0) ccw
  arc A101 (6.0896, 25.2768) -> (3.6431, 25.7435) centre (0, 0) ccw
  dimension "d53" = 1
  constraints: 200 point on circle, 102 centre point, 300 other
  measures "d53" radial gap between concentric circles of A50 A51
extrude "Выдавливание10" add sketch "Эскиз12" along normal blind 1.1 contours A51
chamfer "Фаска3" distance 0.8 angle 45 1 edges at (-19.6, 3.9, 0)
equation "\"d25\" = 0.5 * d24"
